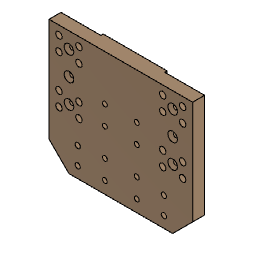
Spindle mount (Autodesk Fusion 360 design; units mm, degrees)
Autodesk Fusion 360 part; units mm, degrees
sketch "Spindle Mount Board" plane through (0, 0, 0) normal (0, 1, 0) x (1, 0, 0)
  line L0 (90, -77.5) -> (-90, -77.5) construction
  line L1 (-90, -77.5) -> (-90, 52.5) construction
  line L2 (-65, 77.5) -> (65, 77.5) construction
  line L3 (90, 52.5) -> (90, -77.5) construction
  line L4 (90, -77.5) -> (-90, 77.5) construction
  line L5 (-90, -77.5) -> (90, 77.5) construction
  line L6 (-90, -77.5) -> (90, -77.5)
  line L7 (90, -77.5) -> (90, 52.5)
  line L8 (90, 52.5) -> (65, 77.5)
  line L9 (90, 52.5) -> (125.7504, 52.5) construction
  line L10 (-90, -77.5) -> (-90, 52.5)
  line L11 (-90, 52.5) -> (-65, 77.5)
  line L12 (-90, 52.5) -> (-54.1427, 52.5) construction
  line L13 (-65, 77.5) -> (65, 77.5)
  line L14 (-77.5, -77.5) -> (-77.5, 25) construction
  line L15 (-52.5, -77.5) -> (-52.5, 25) construction
  line L16 (77.5, -77.5) -> (77.5, 25) construction
  line L17 (52.5, -77.5) -> (52.5, 25) construction
  line L18 (-90, -66.5) -> (90, -66.5) construction
  line L19 (-90, -48.5) -> (90, -48.5) construction
  line L20 (-90, -6.5) -> (90, -6.5) construction
  line L21 (-90, 11.5) -> (90, 11.5) construction
  circle A0 centre (-77.5, -66.5) radius 4
  circle A1 centre (77.5, -66.5) radius 4
  circle A2 centre (-52.5, -66.5) radius 4
  circle A3 centre (52.5, -66.5) radius 4
  circle A4 centre (-77.5, -48.5) radius 4
  circle A5 centre (-52.5, -48.5) radius 4
  circle A6 centre (52.5, -48.5) radius 4
  circle A7 centre (77.5, -48.5) radius 4
  circle A8 centre (-77.5, -6.5) radius 4
  circle A9 centre (-52.5, -6.5) radius 4
  circle A10 centre (52.5, -6.5) radius 4
  circle A11 centre (77.5, -6.5) radius 4
  circle A12 centre (-77.5, 11.5) radius 4
  circle A13 centre (-52.5, 11.5) radius 4
  circle A14 centre (52.5, 11.5) radius 4
  circle A15 centre (77.5, 11.5) radius 4
  line L22 (65, -77.5) -> (65, 25) construction
  line L23 (-65, -77.5) -> (-65, 25) construction
  line L24 (-70, -57.5) -> (70, -57.5) construction
  line L25 (-70, -27.5) -> (70, -27.5) construction
  line L26 (-70, 2.5) -> (70, 2.5) construction
  circle A16 centre (-65, -57.5) radius 2.5
  circle A17 centre (-65, -27.5) radius 2.5
  circle A18 centre (-65, 2.5) radius 2.5
  circle A19 centre (65, 2.5) radius 2.5
  circle A20 centre (65, -27.5) radius 2.5
  circle A21 centre (65, -57.5) radius 2.5
  line L27 (-54, 41.5) -> (54, 41.5) construction
  line L28 (54, 41.5) -> (54, 63.5) construction
  line L29 (54, 63.5) -> (-54, 63.5) construction
  line L30 (-54, 63.5) -> (-54, 41.5) construction
  circle A22 centre (-54, 41.5) radius 3.25
  circle A23 centre (-54, 63.5) radius 3.25
  circle A24 centre (54, 41.5) radius 3.25
  circle A25 centre (54, 63.5) radius 3.25
  line L31 (-20, -20.5) -> (20, -20.5) construction
  line L32 (20, -20.5) -> (20, 3.5) construction
  line L33 (20, 3.5) -> (-20, 3.5) construction
  line L34 (-20, 3.5) -> (-20, -20.5) construction
  circle A26 centre (-20, -20.5) radius 3
  circle A27 centre (-20, 3.5) radius 3
  circle A28 centre (20, -20.5) radius 3
  circle A29 centre (20, 3.5) radius 3
  line L35 (-90, -77.5) -> (-40, -77.5)
  line L36 (-40, -77.5) -> (-40, 77.5)
  line L37 (-40, 77.5) -> (-65, 77.5)
  line L38 (-90, 52.5) -> (-90, -77.5)
  line L39 (90, -77.5) -> (40, -77.5)
  line L40 (40, -77.5) -> (40, 77.5)
  line L41 (40, 77.5) -> (65, 77.5)
  line L42 (90, 52.5) -> (90, -77.5)
  line L43 (-20, 38.5) -> (20, 38.5) construction
  line L44 (20, 38.5) -> (20, 62.5) construction
  line L45 (20, 62.5) -> (-20, 62.5) construction
  line L46 (-20, 62.5) -> (-20, 38.5) construction
  circle A30 centre (-20, 38.5) radius 3
  circle A31 centre (20, 38.5) radius 3
  circle A32 centre (-20, 62.5) radius 3
  circle A33 centre (20, 62.5) radius 3
  dimension "d1" = 180
  dimension "d2" = 155
  dimension "d3" = 130
  dimension "d4" = 135
  dimension "d5" = 130
  dimension "d6" = 45
  dimension "d7" = 25
  dimension "d8" = 25
  dimension "d9" = 25
  dimension "d10" = 25
  dimension "d11" = 12.5
  dimension "d12" = 12.5
  dimension "d13" = 25
  dimension "d14" = 25
  dimension "d15" = 11
  dimension "d16" = 18
  dimension "d17" = 18
  dimension "d18" = 42
  dimension "d19" = 8
  dimension "d20" = 8
  dimension "d21" = 8
  dimension "d22" = 8
  dimension "d23" = 8
  dimension "d24" = 8
  dimension "d25" = 8
  dimension "d26" = 8
  dimension "d27" = 8
  dimension "d28" = 8
  dimension "d29" = 8
  dimension "d30" = 8
  dimension "d31" = 8
  dimension "d32" = 8
  dimension "d33" = 8
  dimension "d34" = 8
  dimension "d35" = 25
  dimension "d36" = 25
  dimension "d37" = 30
  dimension "d38" = 30
  dimension "d39" = 20
  dimension "d40" = 5
  dimension "d41" = 5
  dimension "d42" = 5
  dimension "d43" = 5
  dimension "d44" = 5
  dimension "d45" = 5
  dimension "d46" = 108
  dimension "d47" = 22
  dimension "d48" = 54
  dimension "d49" = 14
  dimension "d50" = 6.5
  dimension "d51" = 6.5
  dimension "d52" = 6.5
  dimension "d53" = 6.5
  dimension "d54" = 24
  dimension "d55" = 20
  dimension "d56" = 57
  dimension "d57" = 6
  dimension "d58" = 6
  dimension "d59" = 6
  dimension "d60" = 6
  dimension "d61" = 50
  dimension "d62" = 50
  dimension "d67" = 40
  dimension "d68" = 24
  dimension "d69" = 20
  dimension "d70" = 3
  dimension "d71" = 6
  dimension "d72" = 6
  dimension "d73" = 6
  dimension "d74" = 6
  constraint perpendicular L0 L1
  constraint parallel L0 L2
  constraint parallel L1 L3
  constraint horizontal L0
  constraint coincident L4 origin
  constraint coincident L5 origin
  constraint perpendicular L0 L7
  constraint horizontal L9
  constraint perpendicular L6 L10
  constraint horizontal L12
  constraint coincident L0 L14.start
  constraint perpendicular L6 L14
  constraint coincident L0 L15.start
  constraint perpendicular L0 L15
  constraint coincident L6 L16.start
  constraint perpendicular L0 L16
  constraint coincident L0 L17.start
  constraint perpendicular L0 L17
  constraint coincident L1 L18.start
  constraint coincident L3 L18.end
  constraint coincident L1 L19.start
  constraint coincident L3 L19.end
  constraint coincident L10 L20.start
  constraint coincident L7 L20.end
  constraint coincident L1 L21.start
  constraint coincident L3 L21.end
  constraint perpendicular L10 L18
  constraint perpendicular L1 L19
  constraint perpendicular L1 L20
  constraint perpendicular L10 L21
  constraint coincident L14 A0.centre
  constraint coincident L18 A0.centre
  constraint coincident L16 A1.centre
  constraint coincident L18 A1.centre
  constraint coincident L15 A2.centre
  constraint coincident L18 A2.centre
  constraint coincident L18 A3.centre
  constraint coincident L17 A3.centre
  constraint coincident L14 A4.centre
  constraint coincident L19 A4.centre
  constraint coincident L15 A5.centre
  constraint coincident L19 A5.centre
  constraint coincident L19 A6.centre
  constraint coincident L17 A6.centre
  constraint coincident L16 A7.centre
  constraint coincident L19 A7.centre
  constraint coincident L20 A8.centre
  constraint coincident L14 A8.centre
  constraint coincident L20 A9.centre
  constraint coincident L15 A9.centre
  constraint coincident L17 A10.centre
  constraint coincident L20 A10.centre
  constraint coincident L16 A11.centre
  constraint coincident L20 A11.centre
  constraint coincident L14 A12.centre
  constraint coincident L21 A12.centre
  constraint coincident L15 A13.centre
  constraint coincident L21 A13.centre
  constraint coincident L21 A14.centre
  constraint coincident L17 A14.centre
  constraint coincident L16 A15.centre
  constraint coincident L21 A15.centre
  constraint coincident L0 L22.start
  constraint coincident L0 L23.start
  constraint perpendicular L0 L22
  constraint perpendicular L0 L23
  constraint perpendicular L22 L24
  constraint perpendicular L22 L25
  constraint perpendicular L22 L26
  constraint coincident L24 A16.centre
  constraint coincident L23 A16.centre
  constraint coincident L25 A17.centre
  constraint coincident L23 A17.centre
  constraint coincident L26 A18.centre
  constraint coincident L23 A18.centre
  constraint coincident L26 A19.centre
  constraint coincident L22 A19.centre
  constraint coincident L25 A20.centre
  constraint coincident L22 A20.centre
  constraint coincident L24 A21.centre
  constraint coincident L22 A21.centre
  constraint horizontal L27
  constraint vertical L28
  constraint horizontal L29
  constraint vertical L30
  constraint coincident L27.start L30.end
  constraint coincident L29.end L30.start
  constraint coincident L27.end L28.start
  constraint coincident L28.end L29.start
  constraint horizontal L31
  constraint vertical L32
  constraint horizontal L33
  constraint vertical L34
  constraint coincident L31.start L34.end
  constraint coincident L33.end L34.start
  constraint coincident L31.end L32.start
  constraint coincident L32.end L33.start
  constraint horizontal L35
  constraint vertical L36
  constraint horizontal L37
  constraint vertical L38
  constraint horizontal L39
  constraint vertical L40
  constraint horizontal L41
  constraint vertical L42
  constraint horizontal L43
  constraint vertical L44
  constraint horizontal L45
  constraint vertical L46
  constraint coincident L43.start L46.end
  constraint coincident L43.end L44.start
  constraint coincident L45.end L46.start
  constraint coincident L44.end L45.start
  measures "d1" distance of L4.end L5.end
  measures "d2" distance of L0.end L4.end
  measures "d3" distance of L0.start L3.start
  measures "d4" angle of L8 L9
  measures "d5" distance of L0.end L1.end
  measures "d6" angle of L11 L12
  measures "d7" vertical distance of L1.end L2.start
  measures "d8" vertical distance of L3.start L2.end
  measures "d9" horizontal distance of L1.end L2.start
  measures "d10" horizontal distance of L3.start L2.end
  measures "d11" distance of L1 L14
  measures "d12" distance of L7 L16
  measures "d13" distance of L14 L15
  measures "d14" distance of L16 L17
  measures "d15" distance of L6 L18
  measures "d16" distance of L18 L19
  measures "d17" distance of L20 L21
  measures "d18" distance of L19 L20
  measures "d19" diameter of A0
  measures "d20" diameter of A1
  measures "d21" diameter of A2
  measures "d22" diameter of A3
  measures "d23" diameter of A4
  measures "d24" diameter of A5
  measures "d25" diameter of A6
  measures "d26" diameter of A7
  measures "d27" diameter of A8
  measures "d28" diameter of A9
  measures "d29" diameter of A10
  measures "d30" diameter of A11
  measures "d31" diameter of A12
  measures "d32" diameter of A13
  measures "d33" diameter of A14
  measures "d34" diameter of A15
  measures "d35" distance of L1 L23
  measures "d36" distance of L3 L22
  measures "d37" distance of L25 L26
  measures "d38" distance of L24 L25
  measures "d39" distance of L6 L24
  measures "d40" diameter of A16
  measures "d41" diameter of A17
  measures "d42" diameter of A18
  measures "d43" diameter of A19
  measures "d44" diameter of A20
  measures "d45" diameter of A21
  measures "d46" distance of L27.start L27.end
  measures "d47" distance of L27.start L29.end
  measures "d48" distance of origin L28
  measures "d49" distance of L13 L29
  measures "d50" diameter of A22
  measures "d51" diameter of A23
  measures "d52" diameter of A24
  measures "d53" diameter of A25
  measures "d54" distance of L31.start L33.end
  measures "d55" distance of origin L32
  measures "d56" distance of L6 L31
  measures "d57" diameter of A26
  measures "d58" diameter of A27
  measures "d59" diameter of A28
  measures "d60" diameter of A29
  measures "d61" distance of L0.end L35.end
  measures "d62" distance of L0.start L39.end
  measures "d67" distance of L43.start L43.end
  measures "d68" distance of L43.start L45.end
  measures "d69" distance of origin L44
  measures "d70" distance of L27 L43
  measures "d71" diameter of A30
  measures "d72" diameter of A31
  measures "d73" diameter of A32
  measures "d74" diameter of A33
extrude "Extrude3" add sketch "Spindle Mount Board" along normal blind 18 contours L6 L13 L36 L40
extrude "Extrude4" add sketch "Spindle Mount Board" along normal blind 15 contours L6 L10 L11 L13 L35 L36 L37 L38 | L6 L7 L8 L13 L39 L40 L41 L42
extrude "Extrude5" add sketch "Spindle Mount Board" along normal blind 18 contours A30 | A31 | A32 | A33
extrude "Extrude6" cut sketch "Spindle Mount Board" along normal blind 6 contours A30 | A31 | A32 | A33
chamfer "Chamfer1" distance 3.5 angle 45 6 edges at (-67.3308, 0, 56.596) (-67.3308, 0, 26.596) (-67.3308, 0, -3.404) (62.6692, 0, -3.404) (62.6692, 0, 26.596) (62.6692, 0, 56.596)
named bodies: "Board"
